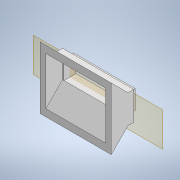
# Autodesk Inventor part: solids hopper
Saved by Autodesk Inventor 2022 (Build 260153000, 153)
## iProperties
Created: 2022-04-23
Part Number: solids hopper
Material: Generic
Document SubType Name: Modeling
Designer: efred
Density: 1 g/cm^3
Appearance: Default
Author: efred
Autodesk Inventor part; units mm, degrees
ref_plane "YZ Plane" through (0, 0, 0) normal (1, 0, 0) x (0, 1, 0)
ref_plane "XZ Plane" through (0, 0, 0) normal (0, 1, 0) x (-1, 0, 0)
ref_plane "XY Plane" through (0, 0, 0) normal (0, 0, 1) x (1, 0, 0)
sketch "Sketch1" plane through (0, 0, 0) normal (0, 0, 1) x (1, 0, 0)
  line L0 (24.7, 6.5) -> (13, 6.5) projected
  line L1 (13, 6.5) -> (13, -1.6) projected
  line L2 (13, -1.6) -> (-13, -1.6) projected
  line L3 (-13, -1.6) -> (-13, 6.5) projected
  line L4 (-13, 6.5) -> (-24.7, 6.5) projected
  line L5 (-24.7, 6.5) -> (-24.7, -6.5) projected
  line L6 (-24.7, -6.5) -> (24.7, -6.5) projected
  line L7 (24.7, -6.5) -> (24.7, 6.5) projected
  line L8 (-24.7, 6.6) -> (24.7, 6.6) projected
  line L9 (24.7, 6.6) -> (24.7, 9.6) projected
  line L10 (-24.7, 9.6) -> (24.7, 9.6) projected
  line L11 (-24.7, 6.6) -> (-24.7, 9.6) projected
  line L12 (-12.9, -1.5) -> (12.9, -1.5)
  line L13 (12.9, -1.5) -> (12.9, 6.5)
  line L14 (12.9, 6.5) -> (-12.9, 6.5)
  line L15 (-12.9, 6.5) -> (-12.9, -1.5)
  line L16 (11.9, -0.5) -> (-11.9, -0.5)
  line L17 (-11.9, -0.5) -> (-11.9, 5.5)
  line L18 (-11.9, 5.5) -> (11.9, 5.5)
  line L19 (11.9, 5.5) -> (11.9, -0.5)
  point P0 (0, 0)
  dimension "d0" = 0.1
  dimension "d1" = 0.1
  dimension "d2" = 0.1
  dimension "d3" = 0.1
  dimension "d4" = 1
  constraints: 16 end point, 4 parallel, 2 perpendicular, 1 horizontal, 3 other
  measures "d0" distance between parallel lines of L8 L14
  measures "d1" distance between parallel lines of L2 L12
  measures "d2" distance between parallel lines of L3 L15
  measures "d3" distance between parallel lines of L1 L13
  measures "d4" distance between parallel lines of L12 L16
extrude "Extrusion1" add sketch "Sketch1" along normal mid plane 5 contours L15 L14 L13 L12
ref_plane "Work Plane1" through (0, 0, 0.1) normal (0, 0, 1) x (1, 0, 0)
sketch "Sketch2" plane through (0, 0, 0.1) normal (0, 0, 1) x (1, 0, 0)
  line L0 (12.9, -1.5) -> (12.9, 6.5) projected
  line L1 (12.9, 6.5) -> (-12.9, 6.5) projected
  line L2 (-12.9, 6.5) -> (-12.9, -1.5) projected
  line L3 (-12.9, -1.5) -> (12.9, -1.5) projected
  line L4 (11.9, -0.5) -> (-11.9, -0.5) projected
  line L5 (-11.9, -0.5) -> (-11.9, 5.5) projected
  line L6 (-11.9, 5.5) -> (11.9, 5.5) projected
  line L7 (11.9, 5.5) -> (11.9, -0.5) projected
  line L8 (-14.9, -3.5) -> (-14.9, 8.5)
  line L9 (-14.9, 8.5) -> (14.9, 8.5)
  line L10 (14.9, 8.5) -> (14.9, -3.5)
  line L11 (14.9, -3.5) -> (-14.9, -3.5)
  point P0 (0, 0)
  dimension "d7" = 2
  constraints: 8 end point, 3 other
  measures "d7" distance between parallel lines of L2 L8
extrude "Extrusion2" add sketch "Sketch2" along normal up to surface (2.4 mm away) contours L8 L9 L10 L11
sketch "Sketch3" plane through (0, 0, 0) normal (1, 0, 0) x (0, 1, 0)
  line L0 (5.5, -2.5) -> (5.5, 2.5) projected
  line L1 (5.5, 2.5) -> (12.5, 9.5)
  line L2 (12.5, 9.5) -> (15.5, 9.5)
  line L3 (8.5, 2.5) -> (-3.5, 2.5) projected
  line L4 (15.5, 9.5) -> (8.5, 2.5)
  line L5 (2.5, 2.5) -> (2.5, -1.8048)
  line L6 (-0.5, 2.5) -> (-7.5, 9.5)
  line L7 (-7.5, 9.5) -> (-10.5, 9.5)
  line L8 (-10.5, 9.5) -> (-3.5, 2.5)
  point P0 (0, 0)
  dimension "d10" = 20
  dimension "d11" = 45
  constraints: 14 end point, 3 symmetric about line, 1 midpoint, 1 parallel, 1 perpendicular, 1 vertical
  measures "d10" distance of L1.end L6.end
  measures "d11" angle of L3 L1
extrude "Extrusion3" add sketch "Sketch3" along normal mid plane 25
sketch "Sketch4" plane through (-12.5, 0, 0) normal (-1, 0, 0) x (0, 0, 1)
  line L0 (9.5, 12.5) -> (9.5, 15.5) projected
  line L1 (9.5, 15.5) -> (2.5, 8.5) projected
  line L2 (2.5, 5.5) -> (2.5, 8.5) projected
  line L3 (2.5, 5.5) -> (9.5, 12.5) projected
  line L4 (2.5, -3.5) -> (2.5, -0.5) projected
  line L5 (2.5, -3.5) -> (9.5, -10.5) projected
  line L6 (9.5, -10.5) -> (9.5, -7.5) projected
  line L7 (9.5, -7.5) -> (2.5, -0.5) projected
  line L8 (2.5, -3.5) -> (2.5, 8.5) projected
  line L9 (9.5, 15.5) -> (9.5, 12.5) projected
  line L10 (9.5, 12.5) -> (9.5, -7.5)
  point P0 (0, 0)
  constraints: 2 end point, 1 collinear
extrude "Extrusion4" add sketch "Sketch4" along normal up to surface (2.4 mm away)
mirror "Mirror1" about plane through (0, 0, 0) normal (1, 0, 0) of "Extrusion4"
body "Solid1"
